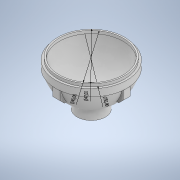
# Autodesk Inventor part: Pommeau globe blanc
Saved by Autodesk Inventor 2021 (Build 250183000, 183)
## iProperties
Created: 2020-09-18
Part Number: Pommeau globe blanc
Material: Générique
Document SubType Name: Modeling
Designer: Utilisateur
Density: 1 g/cm^3
Appearance: Par défaut
Author: Utilisateur
Autodesk Inventor part; units mm, degrees
ref_plane "YZ Plane" through (0, 0, 0) normal (1, 0, 0) x (0, 1, 0)
ref_plane "XZ Plane" through (0, 0, 0) normal (0, 1, 0) x (-1, 0, 0)
ref_plane "XY Plane" through (0, 0, 0) normal (0, 0, 1) x (1, 0, 0)
sketch "Esquisse1" plane through (0, 0, 0) normal (0, 0, 1) x (1, 0, 0)
  circle A0 centre (0, 0) radius 25
  line L0 (0, 28.8291) -> (0, -38.3219)
  line L1 (-31.3088, 0) -> (57.5068, 0)
  arc A1 (22.3616, -25) -> (25, 0) centre (-41.3202, -5.6401) ccw
  line L2 (0, -25) -> (22.3616, -25)
  point P0 (0, 25)
  point P1 (0, -25)
  point P2 (-25, 0)
  dimension "d21" = 50
  constraints: 6 end point, 4 point on circle, 2 centre point, 1 coincident, 1 horizontal, 1 perpendicular, 1 point on line, 1 tangent, 1 vertical
  measures "d21" diameter of A0
revolve "Révolution1" add sketch "Esquisse1" angle 360 about axis through (0, 28.8291, 0) along (0, -1, 0) picked at (16.4577, -1.8543) contours L0 L1 A0
sketch "Esquisse2" plane through (0, 0, 0) normal (1, 0, 0) x (0, 1, 0)
  line L0 (-5, 2.625) -> (-14, 2.625)
  line L1 (-14, 2.625) -> (-14, -2.375)
  line L2 (-14, -2.375) -> (-5, -2.375)
  line L3 (-5, -2.375) -> (-5, 2.625)
  line L4 (-5, 2.625) -> (-14, -2.375) construction
  line L5 (-14, 2.625) -> (-5, -2.375) construction
  line L6 (0, 25) -> (0, -25) projected
  point P0 (0, 0)
  point P1 (-9.5, 0.125)
  dimension "d5" = 9
  dimension "d6" = 5
  dimension "d11" = 5
  constraints: 12 end point, 2 midpoint, 2 parallel, 1 horizontal, 1 perpendicular
  measures "d5" distance of L0.start L0.end
  measures "d6" distance of L2.end L0.start
  measures "d11" distance between parallel lines of L6 L3
extrude "Extrusion1" add sketch "Esquisse2" along normal mid plane 50
sketch "Esquisse3" plane through (0, 0, 0) normal (0, 0, 1) x (1, 0, 0)
  line L0 (-2, -5) -> (3, -5)
  line L1 (3, -5) -> (3, -14)
  line L2 (3, -14) -> (-2, -14)
  line L3 (-2, -14) -> (-2, -5)
  line L4 (-2, -5) -> (3, -14) construction
  line L5 (3, -5) -> (-2, -14) construction
  line L6 (-25, 0) -> (25, 0) projected
  point P0 (0, 0)
  point P1 (0.5, -9.5)
  dimension "d12" = 9
  dimension "d13" = 5
  dimension "d14" = 5
  constraints: 12 end point, 2 midpoint, 2 parallel, 1 horizontal, 1 perpendicular
  measures "d12" distance of L2.end L0.start
  measures "d13" distance of L1.end L2.end
  measures "d14" distance between parallel lines of L6 L0
extrude "Extrusion2" add sketch "Esquisse3" along normal mid plane 50
sketch "Esquisse4" plane through (0, 0, 0) normal (0, 1, 0) x (-1, 0, 0)
  circle A0 centre (0, 0) radius 10
  dimension "d23" = 20
  constraints: 1 centre point, 1 coincident
  measures "d23" diameter of A0
extrude "Extrusion3" add sketch "Esquisse4" against normal blind 30
sketch "Esquisse5" plane through (0, -30, 0) normal (0, -1, 0) x (1, 0, 0)
  circle A0 centre (0, 0) radius 9.5
  dimension "d26" = 19
  constraints: 1 centre point, 1 coincident
  measures "d26" diameter of A0
extrude "Trou creux extrusion" cut sketch "Esquisse5" against normal blind 35
sketch "Esquisse6" plane through (0, 0, 0) normal (1, 0, 0) x (0, 1, 0)
  line L0 (0, 25) -> (0, -25) projected
  arc A0 (0, 22.5) -> (0, -22.5) centre (0, 0) ccw
  line L1 (0, -22.5) -> (0, 22.5)
  line L2 (15.0962, 0) -> (-32.1154, 0)
  point P0 (-22.5, 0)
  point P1 (0, -22.5)
  dimension "d32" = 22.5
  constraints: 4 end point, 2 point on circle, 1 centre point, 1 coincident, 1 collinear, 1 horizontal, 1 point on line
  measures "d32" distance of A0.centre L1.start
revolve "Creuse Révolution" cut sketch "Esquisse6" angle 360 about axis through (0, 15.0962, 0) along (0, -1, 0) picked at (-1.6689, -14.812) contours L0 A0 L2
sketch "Esquisse9" plane through (0, 0, 0) normal (1, 0, 0) x (0, 1, 0)
  line L0 (-5, 25) -> (-14, 25) projected
  line L1 (-5, 25) -> (0, 25)
  line L2 (0, 25) -> (0, 23.5)
  line L3 (0, 25) -> (0, -25) projected
  arc A0 (-5, 24.4131) -> (-14, 20.6155) centre (0, 0) ccw projected
  line L4 (-5, 24.4131) -> (-5, 25) projected
  line L5 (-5, 24.4131) -> (-5, 25)
  line L6 (23.4968, 0) -> (-36.2187, 0)
  point P0 (0, 0)
  dimension "d37" = 1.5
  dimension "d38" = 5
  constraints: 8 end point, 2 horizontal, 1 point on line, 1 vertical
  measures "d37" distance of L1.end L2.end
  measures "d38" distance of L0.start L1.end
revolve "Grand révolution cylindre" add sketch "Esquisse9" angle 360 about axis through (0, 23.4968, 0) along (0, -1, 0) fills toward (-4.95, 24.7066) open curves L5 L1 L2
sketch "Esquisse11" plane through (0, 0, 0) normal (0, 0, 1) x (1, 0, 0)
  line L0 (23.5, 0) -> (23.5, 2)
  line L1 (23.5, 2) -> (22.5, 2)
  line L2 (-22.5, 0) -> (22.5, 0) projected
  line L3 (22.5, 2) -> (22.5, 0)
  line L4 (23.5, 0) -> (22.5, 0)
  line L5 (-25, 0) -> (25, 0) projected
  line L6 (0, 21.1238) -> (0, -40.5241)
  point P0 (0, 0)
  dimension "d46" = 1
  dimension "d53" = 2
  constraints: 10 end point, 2 perpendicular, 2 vertical, 1 collinear
  measures "d46" distance of L0.end L1.end
  measures "d53" distance of L0.start L0.end
revolve "Moyenne révolution dernier cylindre" add sketch "Esquisse11" angle 360 about axis through (0, 21.1238, 0) along (0, -1, 0)
chamfer "Chanfrein1" distance 3 angle 45 4 edges at (0.5, -14, 25) (25, -14, 0.125) (-25, -14, 0.125) (0.5, -14, -25)
